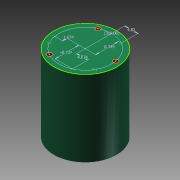
# Autodesk Inventor part: Connector_PCB
Saved by Autodesk Inventor 2011 SP2 (Build 150309200, 309)
## iProperties
Created: 2012-03-06
Part Number: Connector_PCB
Document SubType Name: Modeling
Designer: sungwook
Density: 1 g/cm^3
Author: sungwook
Autodesk Inventor part; units mm, degrees
ref_plane "YZ Plane" through (0, 0, 0) normal (1, 0, 0) x (0, 1, 0)
ref_plane "XZ Plane" through (0, 0, 0) normal (0, 1, 0) x (-1, 0, 0)
ref_plane "XY Plane" through (0, 0, 0) normal (0, 0, 1) x (1, 0, 0)
sketch "Sketch1" plane through (0, 0, 0) normal (0, 0, 1) x (1, 0, 0)
  circle A0 centre (0, 0) radius 11.5
  dimension "d0" = 23
  constraints: 1 centre point, 1 coincident
  measures "d0" diameter of A0
extrude "Extrusion1" add sketch "Sketch1" along normal blind 28
sketch "Sketch2" plane through (0, 0, 28) normal (0, 0, 1) x (1, 0, 0)
  circle A0 centre (0, 0) radius 11.5 projected
  line L0 (0, -16.1) -> (0, 16.1) projected
  line L1 (-16.1, 0) -> (16.1, 0) projected
  point P0 (0, 9.69)
  point P1 (-8.3918, -4.845)
  point P2 (8.3918, -4.845)
  point P3 (-4.074, 8.737)
  point P4 (-4.82, -8.349)
  point P5 (9.494, 1.674)
  dimension "d3" = 9.69
  dimension "d6" = 360
  dimension "d8" = 8.737
  dimension "d9" = 4.074
  dimension "d10" = 4.82
  dimension "d11" = 8.349
  dimension "d12" = 9.494
  dimension "d13" = 1.674
  constraints: 1 point on line, 4 other
  measures "d3" distance from line of L1 point (0, 9.69)
  measures "d8" vertical distance of A0.centre point (-4.074, 8.737)
  measures "d9" distance from line of L0 point (-4.074, 8.737)
  measures "d10" distance from line of L0 point (-4.82, -8.349)
  measures "d11" vertical distance of A0.centre point (-4.82, -8.349)
  measures "d12" distance from line of L0 point (9.494, 1.674)
  measures "d13" vertical distance of A0.centre point (9.494, 1.674)
hole "Hole1" at (-4.074, 8.737, 28) at (-4.82, -8.349, 28) at (9.494, 1.674, 28) direction (0, 0, -1) diameter 1.778 end through all clearance for "Flat Head Machine Screw (82)" size "#0" standard "Ansi Unified Screw Threads"
sketch "Sketch3" plane through (0, 0, 28) normal (0, 0, 1) x (1, 0, 0)
  circle A0 centre (9.494, 1.674) radius 0.889 projected
  circle A1 centre (-4.82, -8.349) radius 0.889 projected
  circle A2 centre (-4.074, 8.737) radius 0.889 projected
  circle A3 centre (0, 0) radius 11.5 projected
  circle A4 centre (0, 0) radius 11.5
  point P0 (0, 9.69)
  point P1 (-8.3918, -4.845)
  point P2 (8.3918, -4.845)
  point P3 (4.074, -8.737)
  point P4 (4.82, 8.349)
  point P5 (-9.494, -1.674)
  dimension "d23" = 360
  dimension "d24" = -8.737
  dimension "d25" = 8.349
  dimension "d26" = 1.674
  dimension "d27" = 4.074
  dimension "d28" = 4.82
  constraints: 1 centre point, 1 other
  measures "d24" vertical distance of A4.centre point (4.074, -8.737)
  measures "d25" vertical distance of A4.centre point (4.82, 8.349)
  measures "d26" vertical distance of A4.centre point (-9.494, -1.674)
  measures "d27" horizontal distance of point (4.074, -8.737) A3.centre
  measures "d28" horizontal distance of A3.centre point (4.82, 8.349)
body "Solid1"
